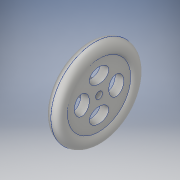
# Autodesk Inventor part: Fake Rad
Saved by Autodesk Inventor 2018 (Build 220112000, 112)
## iProperties
Created: 2019-03-04
Part Number: Fake Rad
Material: Aluminium 6061
Document SubType Name: Modeling
Designer: RedBots
Density: 2.82337 g/cm^3
Appearance: Aluminium - flach
Mass: 30 g
Surface Area: 52.7483 cm^2
Volume: 10.6256 cm^3
Author: RedBots
Autodesk Inventor part; units mm, degrees
ref_plane "YZ Plane" through (0, 0, 0) normal (1, 0, 0) x (0, 1, 0)
ref_plane "XZ Plane" through (0, 0, 0) normal (0, 1, 0) x (-1, 0, 0)
ref_plane "XY Plane" through (0, 0, 0) normal (0, 0, 1) x (1, 0, 0)
sketch "Skizze1" plane through (0, 0, 0) normal (0, 0, 1) x (1, 0, 0)
  line L0 (0, 0) -> (5, 0)
  line L1 (5, 0) -> (5, 21.5)
  line L2 (5, 21.5) -> (0, 21.5)
  line L3 (0, 21.5) -> (0, 0)
  circle A0 centre (2.5, 21.5) radius 4
  line L4 (0, 0) -> (-7, 0)
  line L5 (-7, 0) -> (-7, 5)
  line L6 (-7, 5) -> (0, 5)
  line L7 (0, 5) -> (0, 0)
  line L8 (2.45, 25.5) -> (2.55, 25.5)
  line L9 (2.5, 21.5) -> (2.5, 25.5) construction
  line L10 (2.45, 25.5) -> (2.45, 25.4997)
  line L11 (2.55, 25.5) -> (2.55, 25.4997)
  dimension "d0" = 8
  dimension "d1" = 21.5
  dimension "d2" = 5
  dimension "d3" = 7
  dimension "d4" = 5
  dimension "d9" = 0.1
  constraints: 24 end point, 4 parallel, 3 horizontal, 3 point on circle, 3 vertical, 2 midpoint, 2 perpendicular, 1 centre point
  measures "d0" diameter of A0
  measures "d1" distance of L0.end L1.end
  measures "d2" distance of L0.start L0.end
  measures "d3" distance of L5.end L6.end
  measures "d4" distance of L4.end L5.end
  measures "d9" distance of L8.start L8.end
revolve "Umdrehung1" add sketch "Skizze1" angle 360 about axis through (0, 0, 0) along (1, 0, 0)
sketch "Skizze2" plane through (-7, 0, 0) normal (-1, 0, 0) x (0, 0, 1)
  circle A0 centre (0, 0) radius 2
  dimension "d6" = 4
  constraints: 1 centre point, 1 coincident
  measures "d6" diameter of A0
extrude "Extrusion1" cut sketch "Skizze2" against normal up to next
sketch "Skizze3" plane through (5, 0, 0) normal (1, 0, 0) x (0, 0, -1)
  line L0 (0, 0) -> (-10, 0) construction
  ellipse E0 centre (-10, 0) end of major axis (-10, 5.6146) minor radius 4.3356
  ellipse E1 centre (0, -10) end of major axis (-5.6146, -10) minor radius 4.3356
  ellipse E2 centre (10, 0) end of major axis (10, -5.6146) minor radius 4.3356
  ellipse E3 centre (0, 10) end of major axis (5.6146, 10) minor radius 4.3356
  dimension "d10" = 10
  dimension "d13" = 360
  constraints: 2 end point, 1 coincident, 1 horizontal, 17 other
  measures "d10" distance of L0.start L0.end
extrude "Extrusion2" cut sketch "Skizze3" against normal up to next
